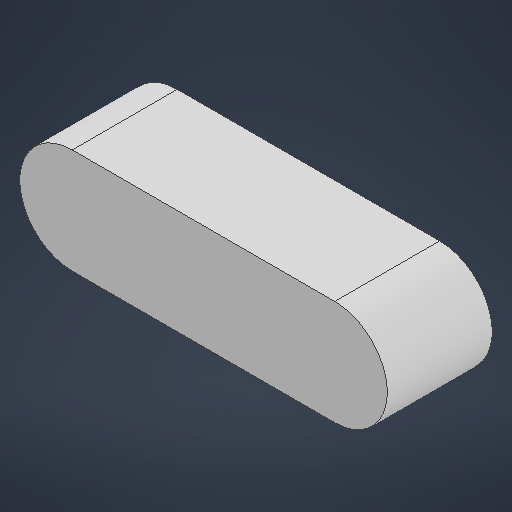
# Autodesk Inventor part: Part1
Saved by Autodesk Inventor 2026.2 (Build 302298010, 298A)
## iProperties
Created: 2026-04-16
Part Number: Part1
Material: Generic
Document SubType Name: Modeling
Designer: mrcm
Density: 1 g/cm^3
Appearance: Default
Author: mrcm
Autodesk Inventor part; units mm, degrees
ref_plane "YZ Plane" through (0, 0, 0) normal (1, 0, 0) x (0, 1, 0)
ref_plane "XZ Plane" through (0, 0, 0) normal (0, 1, 0) x (-1, 0, 0)
ref_plane "XY Plane" through (0, 0, 0) normal (0, 0, 1) x (1, 0, 0)
sketch "Sketch1" plane through (0, 0, 0) normal (0, 0, 1) x (1, 0, 0)
  line L0 (-25, 0) -> (25, 0) construction
  line L1 (-25, -10) -> (25, -10)
  line L2 (25, 10) -> (-25, 10)
  arc A0 (-25, 10) -> (-25, -10) centre (-25, 0) ccw
  arc A1 (25, -10) -> (25, 10) centre (25, 0) ccw
  point P0 (0, 0)
  dimension "d0" = 10
  dimension "d1" = 50
  constraints: 8 end point, 4 point on circle, 4 tangent, 2 centre point, 1 horizontal, 1 midpoint, 1 parallel
  measures "d0" radius of A1
  measures "d1" distance of L0.end L0.start
extrude "Extrusion1" add sketch "Sketch1" along normal blind 20
body "Solid1"
